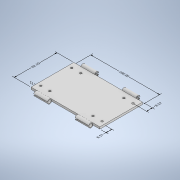
# Autodesk Inventor part: Part2
Saved by Autodesk Inventor 2020 (Build 240168000, 168)
## iProperties
Created: 2019-08-08
Part Number: Part2
Material: Generic
Document SubType Name: Modeling
Designer: Nicolas
Density: 1 g/cm^3
Appearance: Default
Author: Nicolas
Autodesk Inventor part; units mm, degrees
ref_plane "YZ Plane" through (0, 0, 0) normal (1, 0, 0) x (0, 1, 0)
ref_plane "XZ Plane" through (0, 0, 0) normal (0, 1, 0) x (-1, 0, 0)
ref_plane "XY Plane" through (0, 0, 0) normal (0, 0, 1) x (1, 0, 0)
sketch "Sketch1" plane through (0, 0, 0) normal (1, 0, 0) x (0, 1, 0)
  line L0 (0.3153, 51.2567) -> (-2.5847, 51.2567)
  line L1 (-2.5847, 51.2567) -> (-2.5847, -10.8433)
  line L2 (-2.5847, -10.8433) -> (0.3153, -10.8433)
  line L3 (0.3153, -10.8433) -> (0.3153, 51.2567)
  arc A0 (0.3153, 51.2567) -> (-0.0756, 57.3616) centre (-1.1163, 54.23) ccw
  arc A1 (-2.2756, 57.3196) -> (-2.5847, 51.2567) centre (-1.1371, 54.2222) ccw
  line L4 (-2.2756, 57.3196) -> (-2.2756, 56.2196)
  line L5 (-0.0756, 57.3616) -> (-0.0756, 56.2616)
  arc A2 (-2.2756, 56.2196) -> (-0.0756, 56.2616) centre (-1.1371, 54.2222) ccw
  arc A3 (-2.5847, -10.8433) -> (-2.5847, -16.9063) centre (-1.2354, -13.8748) ccw
  arc A4 (-0.3847, -16.0719) -> (-2.5847, -15.8063) centre (-1.2354, -13.8748) ccw
  arc A5 (-0.3847, -17.1719) -> (0.3153, -10.8433) centre (-1.2354, -13.8748) ccw
  line L6 (-2.5847, -15.8063) -> (-2.5847, -16.9063)
  line L7 (-0.3847, -16.0719) -> (-0.3847, -17.1719)
  point P0 (0, 0)
  dimension "d0" = 2.9
  dimension "d1" = 62.1
  dimension "d163" = 1.1
  dimension "d164" = 1.1
  dimension "d165" = 2.2
  dimension "d166" = 2.2991
  dimension "d167" = 3.3
  dimension "d168" = 3.3
  dimension "d171" = 6.063
  dimension "d172" = 6.1049
  dimension "d174" = 6.063
  dimension "d176" = 1.1
  dimension "d177" = 1.1
  dimension "d178" = 2.2
  constraints: 16 end point, 13 point on circle, 6 centre point, 4 vertical, 3 coincident, 2 parallel, 2 point on line, 1 horizontal, 1 perpendicular
  measures "d0" distance between parallel lines of L1 L3
  measures "d1" distance between parallel lines of L2 L0
  measures "d163" distance of L4.start L4.end
  measures "d164" distance of L5.start L5.end
  measures "d165" distance between parallel lines of L5 L4
  measures "d166" radius of A2
  measures "d167" radius of A1
  measures "d168" radius of A0
  measures "d171" vertical distance of L4.start L0.end
  measures "d172" vertical distance of L5.start L0.start
  measures "d174" distance of L1.end L6.end
  measures "d176" distance of L6.end L6.start
  measures "d177" distance of L7.end L7.start
  measures "d178" horizontal distance of L7.end L6.end
extrude "Extrusion1" add sketch "Sketch1" against normal blind 20
sketch "Sketch3" plane through (0, 0, 0) normal (1, 0, 0) x (0, 0, -1)
  line L0 (10.8433, -2.5847) -> (-51.2567, -2.5847)
  line L1 (-51.2567, 0.3153) -> (10.8433, 0.3153)
  line L2 (10.8433, 0.3153) -> (10.8433, -2.5847)
  line L3 (10.8433, -2.5847) -> (-51.2567, -2.5847)
  line L4 (-51.2567, -2.5847) -> (-51.2567, 0.3153)
  point P0 (0, 0)
  constraints: 10 end point, 2 parallel, 1 horizontal, 1 perpendicular
extrude "Extrusion2" add sketch "Sketch3" along normal blind 40
sketch "Sketch4" plane through (40, 0, 0) normal (1, 0, 0) x (0, 0, -1)
  line L0 (10.8433, -2.5847) -> (-51.2567, -2.5847)
  line L1 (10.8433, -2.5847) -> (-51.2567, -2.5847)
  line L2 (-51.2567, -2.5847) -> (-51.2567, 0.3153)
  line L3 (-51.2567, 0.3153) -> (10.8433, 0.3153)
  line L4 (10.8433, 0.3153) -> (10.8433, -2.5847)
  arc A0 (-57.3196, -2.2756) -> (-51.2567, -2.5847) centre (-54.2222, -1.1371) ccw
  arc A1 (-57.3196, -2.2756) -> (-51.2567, -2.5847) centre (-54.2222, -1.1371) ccw
  arc A2 (-51.2567, 0.3153) -> (-57.3616, -0.0756) centre (-54.23, -1.1163) ccw
  arc A3 (-51.2567, 0.3153) -> (-57.3616, -0.0756) centre (-54.2286, -1.1372) ccw
  arc A4 (-56.2196, -2.2756) -> (-56.2616, -0.0756) centre (-54.2222, -1.1371) ccw
  arc A5 (-56.2196, -2.2756) -> (-56.2616, -0.0756) centre (-54.2286, -1.1372) ccw
  line L5 (-56.2196, -2.2756) -> (-57.3196, -2.2756)
  line L6 (-56.2196, -2.2756) -> (-57.3196, -2.2756)
  line L7 (-57.3616, -0.0756) -> (-56.2616, -0.0756)
  line L8 (-56.2616, -0.0756) -> (-57.3616, -0.0756)
  arc A6 (-57.3196, -2.2756) -> (-51.2567, -2.5847) centre (-54.2222, -1.1371) ccw
  line L9 (-51.2567, -2.5847) -> (-51.2567, 0.3153)
  arc A7 (-51.2567, 0.3153) -> (-57.3616, -0.0756) centre (-54.23, -1.1163) ccw
  arc A8 (-56.2196, -2.2756) -> (-56.2616, -0.0756) centre (-54.2222, -1.1371) ccw
  line L10 (-57.3196, -2.2756) -> (-56.2196, -2.2756)
  line L11 (-56.2616, -0.0756) -> (-57.3616, -0.0756)
  line L12 (-56.2616, -0.0756) -> (-57.3616, -0.0756)
  line L13 (-56.2616, -0.0756) -> (-57.3616, -0.0756)
  arc A9 (10.8433, -2.5847) -> (16.9063, -2.5847) centre (13.8748, -1.2354) ccw
  arc A10 (10.8433, -2.5847) -> (16.9063, -2.5847) centre (13.8748, -1.2354) ccw
  arc A11 (17.1719, -0.3847) -> (10.8433, 0.3153) centre (13.8748, -1.2354) ccw
  arc A12 (17.1719, -0.3847) -> (10.8433, 0.3153) centre (13.8748, -1.2354) ccw
  arc A13 (16.0719, -0.3847) -> (15.8063, -2.5847) centre (13.8748, -1.2354) ccw
  arc A14 (16.0719, -0.3847) -> (15.8063, -2.5847) centre (13.8748, -1.2354) ccw
  line L14 (15.8063, -2.5847) -> (16.9063, -2.5847)
  line L15 (16.0719, -0.3847) -> (17.1719, -0.3847)
  constraints: 32 end point, 30 point on circle, 15 centre point, 7 equal length, 4 concentric, 3 horizontal, 2 coincident, 1 perpendicular
extrude "Extrusion3" add sketch "Sketch4" along normal blind 20 contours L0 L2 L3 L4 | L4 A11 L15 A13 L14 A9 | A0 L5 A4 L7 A3 L2 | A3 A2
sketch "Sketch9" plane through (0, -2.5847, 51.2567) normal (0, 0, 1) x (1, 0, 0)
  line L0 (0, 2.9) -> (40, 2.9) projected
  line L1 (0, 2.9) -> (40, 2.9)
  line L2 (40, 2.9) -> (40, 0)
  line L3 (40, 0) -> (0, 0)
  line L4 (0, 0) -> (0, 2.9)
  point P0 (0, 2.5847)
  constraints: 8 end point, 2 parallel, 1 horizontal, 1 perpendicular
extrude "Extrusion4" add sketch "Sketch9" along normal blind 0.001
sketch "Sketch10" plane through (-20, 0, 0) normal (-1, 0, 0) x (0, 0, 1)
  arc A0 (51.2567, -2.5847) -> (57.3196, -2.2756) centre (54.2222, -1.1371) ccw
  line L0 (-10.8433, 0.3153) -> (-10.8433, -2.5847)
  line L1 (51.2567, -2.5847) -> (-10.8433, -2.5847)
  line L2 (-10.8433, -2.5847) -> (-10.8433, 0.3153)
  line L3 (-10.8433, 0.3153) -> (51.2567, 0.3153)
  line L4 (51.2567, 0.3153) -> (51.2567, -2.5847)
  point P0 (0, 0)
  point P1 (-10.8433, -2.5847)
  constraints: 10 end point, 2 parallel, 2 point on circle, 1 centre point, 1 horizontal, 1 perpendicular
extrude "Extrusion5" add sketch "Sketch10" along normal blind 10
sketch "Sketch11" plane through (60, 0, 0) normal (1, 0, 0) x (0, 0, -1)
  line L0 (10.8433, -2.5847) -> (10.8433, 0.3153)
  arc A0 (-51.2567, 0.3153) -> (-57.3616, -0.0756) centre (-54.23, -1.1163) ccw
  line L1 (10.8433, -2.5847) -> (-51.2567, -2.5847)
  line L2 (-51.2567, -2.5847) -> (-51.2567, 0.3153)
  line L3 (-51.2567, 0.3153) -> (10.8433, 0.3153)
  line L4 (10.8433, 0.3153) -> (10.8433, -2.5847)
  point P0 (0, 0)
  point P1 (-57.2033, 0.3153)
  point P2 (10.8433, 0.3153)
  constraints: 10 end point, 2 parallel, 2 point on circle, 1 centre point, 1 horizontal, 1 perpendicular
extrude "Extrusion6" add sketch "Sketch11" along normal blind 10
sketch "Sketch12" plane through (0, -2.5847, 57.2567) normal (0, -1, 0) x (1, 0, 0)
  line L0 (-20, -6) -> (-30, -6)
  line L1 (-30, -68.1) -> (-30, -6)
  point P0 (-24.59, -14.57)
  dimension "d133" = 8.57
  dimension "d134" = 5.41
  constraints: 4 end point
  measures "d133" distance from line of L0 point (-24.59, -14.57)
  measures "d134" distance from line of L1 point (-24.59, -14.57)
hole "Hole5" at (-24.59, -2.5847, 42.6867) direction (0, 1, 0) diameter 2.921 end through all
sketch "Sketch13" plane through (0, -2.5847, 57.2567) normal (0, -1, 0) x (1, 0, 0)
  line L0 (0, -6) -> (-20, -6)
  circle A0 centre (-24.59, -14.57) radius 1.4605
  point P0 (-11.33, -14.57)
  dimension "d135" = 8.57
  dimension "d136" = 13.26
  constraints: 2 end point, 1 centre point
  measures "d135" distance from line of L0 point (-11.33, -14.57)
  measures "d136" distance of point (-11.33, -14.57) A0.centre
hole "Hole6" at (-11.33, -2.5847, 42.6867) direction (0, 1, 0) diameter 2.921 end through all
sketch "Sketch14" plane through (0, -2.5847, 57.2567) normal (0, -1, 0) x (1, 0, 0)
  line L0 (-30, -68.1) -> (-30, -6) projected
  circle A0 centre (-24.59, -14.57) radius 1.4605 projected
  point P0 (0, -57.2567)
  point P1 (-24.59, -59.53)
  dimension "d137" = 5.41
  dimension "d138" = 44.96
  measures "d137" distance from line of L0 point (-24.59, -59.53)
  measures "d138" distance of point (-24.59, -59.53) A0.centre
hole "Hole7" at (-24.59, -2.5847, -2.2733) direction (0, 1, 0) diameter 2.921 end through all
sketch "Sketch15" plane through (0, -2.5847, 57.2567) normal (0, -1, 0) x (1, 0, 0)
  circle A0 centre (-11.33, -14.57) radius 1.4605 projected
  circle A1 centre (-24.59, -59.53) radius 1.4605 projected
  point P0 (0, -57.2567)
  point P1 (-11.33, -59.53)
  dimension "d139" = 44.96
  dimension "d148" = 13.26
  measures "d139" distance of A0.centre point (-11.33, -59.53)
  measures "d148" distance of point (-11.33, -59.53) A1.centre
hole "Hole8" at (-11.33, -2.5847, -2.2733) direction (0, 1, 0) diameter 2.921 end through all
sketch "Sketch17" plane through (0, -2.5847, 57.2567) normal (0, -1, 0) x (1, 0, 0)
  line L0 (70, -6) -> (70, -68.1) projected
  line L1 (60, -6) -> (70, -6) projected
  point P0 (0, -57.2567)
  point P1 (64.59, -14.57)
  dimension "d142" = 5.41
  dimension "d147" = 8.57
  measures "d142" distance from line of L0 point (64.59, -14.57)
  measures "d147" distance from line of L1 point (64.59, -14.57)
hole "Hole10" at (64.59, -2.5847, 42.6867) direction (0, 1, 0) diameter 2.921 end through all
sketch "Sketch16" plane through (0, -2.5847, 57.2567) normal (0, -1, 0) x (1, 0, 0)
  circle A0 centre (64.59, -14.57) radius 1.4605 projected
  line L0 (40, -6) -> (60, -6) projected
  point P0 (0, -57.2567)
  point P1 (51.33, -14.57)
  dimension "d144" = 13.26
  dimension "d146" = 8.57
  measures "d144" distance of A0.centre point (51.33, -14.57)
  measures "d146" distance from line of L0 point (51.33, -14.57)
hole "Hole9" at (51.33, -2.5847, 42.6867) direction (0, 1, 0) diameter 2.921 end through all
sketch "Sketch19" plane through (0, -2.5847, 57.2567) normal (0, -1, 0) x (1, 0, 0)
  circle A0 centre (64.59, -14.57) radius 1.4605 projected
  line L0 (70, -6) -> (70, -68.1) projected
  point P0 (0, -57.2567)
  point P1 (64.59, -59.53)
  dimension "d141" = 44.96
  dimension "d143" = 5.41
  measures "d141" distance of A0.centre point (64.59, -59.53)
  measures "d143" distance from line of L0 point (64.59, -59.53)
hole "Hole12" at (64.59, -2.5847, -2.2733) direction (0, 1, 0) diameter 2.921 end through all
sketch "Sketch18" plane through (0, -2.5847, 57.2567) normal (0, -1, 0) x (1, 0, 0)
  circle A0 centre (51.33, -14.57) radius 1.4605 projected
  circle A1 centre (64.59, -59.53) radius 1.4605 projected
  point P0 (0, -57.2567)
  point P1 (51.33, -59.53)
  dimension "d140" = 44.96
  dimension "d145" = 13.26
  measures "d140" distance of point (51.33, -59.53) A0.centre
  measures "d145" distance of A1.centre point (51.33, -59.53)
hole "Hole11" at (51.33, -2.5847, -2.2733) direction (0, 1, 0) diameter 2.921 end through all
body "Solid1"
